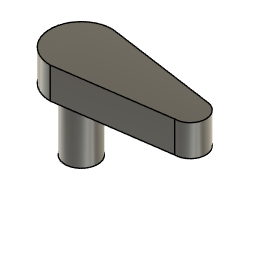
Mecanismo Flipper v1 (Autodesk Fusion 360 archive; units mm, degrees)
design "Flipper"
Autodesk Fusion 360 part; units mm, degrees
sketch "Boceto1" plane through (0, 0, 0) normal (0, 0, 1) x (1, 0, 0)
  circle A0 centre (0, 0) radius 10.5
  dimension "d1" = 21
  constraint coincident A0.centre origin
  measures "d1" diameter of A0
extrude "Extruir1" add sketch "Boceto1" along normal blind 40
sketch "Boceto2" plane through (0, 0, 40) normal (0, 0, 1) x (-1, 0, 0)
  circle A0 centre (0, 0) radius 10.5
  circle A1 centre (0, 0) radius 20
  line L0 (20, 0) -> (-80, 0)
  circle A2 centre (-70, 0) radius 10
  line L1 (0, -20) -> (-70, -10)
  line L2 (-70, 10) -> (0, 20)
  dimension "d4" = 40
  dimension "d5" = 100
  constraint coincident A0.centre A1.centre
  constraint coincident A1 L0.start
  constraint horizontal L0
  constraint coincident L0.end A2
  constraint coincident A1 L1.start
  constraint coincident A2 L1.end
  constraint coincident A2 L2.start
  constraint coincident A1 L2.end
  measures "d4" diameter of A1
  measures "d5" distance of L0.start L0.end
extrude "Extruir2" add sketch "Boceto2" along normal blind 20 contours A0 L0 | A0 A1 L0 L1 | A0 A1 L0 L2 | A0 L0 | A1 L0 A2 L2 | A1 L0 A2 L1 | L0 A2 | L0 A2

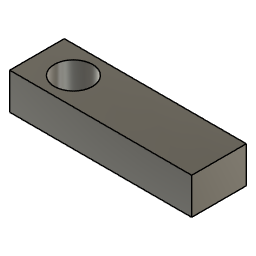
design "Accionador Flipper"
Autodesk Fusion 360 part; units mm, degrees
sketch "Boceto1" plane through (0, 0, 0) normal (0, 0, 1) x (1, 0, 0)
  line L0 (0, 0) -> (100, 0)
  line L1 (100, 0) -> (100, 30)
  line L2 (100, 30) -> (0, 30)
  line L3 (0, 30) -> (0, 0)
  circle A0 centre (20, 15) radius 10.5
  dimension "d1" = 100
  dimension "d2" = 30
  dimension "d3" = 21
  constraint horizontal L0
  constraint vertical L1
  constraint horizontal L2
  constraint vertical L3
  constraint coincident L0.start L3.end
  measures "d1" distance of L0.start L0.end
  measures "d2" distance of L0.start L2.end
  measures "d3" diameter of A0
extrude "Extruir1" add sketch "Boceto1" along normal blind 20
